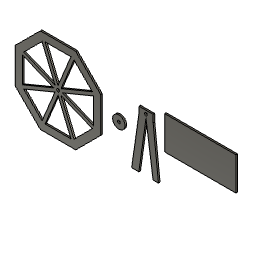
FerrisWheel2 v0 (Autodesk Fusion 360 design; units mm, degrees)
Autodesk Fusion 360 part; units mm, degrees
sketch "Sketch1" plane through (0, 0, 0) normal (0, 1, 0) x (1, 0, 0)
  line L0 (100, -41.4214) -> (100, 41.4213)
  line L1 (100, 41.4213) -> (41.4214, 100)
  line L2 (41.4214, 100) -> (-41.4213, 100)
  line L3 (-41.4213, 100) -> (-100, 41.4214)
  line L4 (-100, 41.4214) -> (-100, -41.4213)
  line L5 (-100, -41.4213) -> (-41.4214, -100)
  line L6 (-41.4214, -100) -> (41.4213, -100)
  line L7 (41.4213, -100) -> (100, -41.4214)
  line L8 (-96.5734, -44.848) -> (-100.1089, -41.3124) construction
  line L9 (-100.1089, -41.3124) -> (-100, -36.3136) construction
  line L10 (-41.4214, -100) -> (-36.4214, -100)
  line L11 (-41.4214, -100) -> (-44.9569, -96.4644)
  line L12 (-100, 41.4214) -> (-100, 36.4214)
  line L13 (-100, 41.4214) -> (-96.4644, 44.9569)
  line L14 (-41.4213, 100) -> (-36.4213, 100)
  line L15 (-41.4213, 100) -> (-44.9569, 96.4645)
  line L16 (41.4214, 100) -> (44.9569, 96.4644)
  line L17 (41.4214, 100) -> (36.4214, 100)
  line L18 (100, 41.4213) -> (100, 36.4213)
  line L19 (100, 41.4213) -> (96.4645, 44.9569)
  line L20 (100, -41.4214) -> (100, -36.4214)
  line L21 (100, -41.4214) -> (96.4644, -44.9569)
  line L22 (41.4213, -100) -> (44.9569, -96.4645)
  line L23 (41.4213, -100) -> (36.4213, -100)
  line L24 (-96.5734, -44.848) -> (100, 36.4213)
  line L25 (96.4645, 44.9569) -> (-100, -36.3136)
  line L26 (-44.9569, -96.4644) -> (36.4214, 100)
  line L27 (44.9569, 96.4644) -> (-36.4214, -100)
  line L28 (36.4213, -100) -> (-44.9569, 96.4645)
  line L29 (-36.4213, 100) -> (44.9569, -96.4645)
  line L30 (96.4644, -44.9569) -> (-100, 36.4214)
  line L31 (-96.4644, 44.9569) -> (100, -36.4214)
  circle A0 centre (0, 0) radius 4
  circle A1 centre (0, 0) radius 17.5
  line L32 (120, 49.7056) -> (49.7056, 120)
  line L33 (49.7056, 120) -> (-49.7056, 120)
  line L34 (-49.7056, 120) -> (-120, 49.7056)
  line L35 (-120, 49.7056) -> (-120, -49.7056)
  line L36 (-120, -49.7056) -> (-49.7056, -120)
  line L37 (-49.7056, -120) -> (49.7056, -120)
  line L38 (49.7056, -120) -> (120, -49.7056)
  line L39 (120, -49.7056) -> (120, 49.7056)
  line L40 (200.3187, 0) -> (200.3187, 150) construction
  line L41 (200.3187, 150) -> (220.3187, 150) construction
  line L42 (200.3187, 150) -> (180.3187, 150) construction
  line L43 (220.3187, 150) -> (235.3187, 150)
  line L44 (220.3187, -10) -> (180.3187, -10)
  line L45 (180.3187, -10) -> (180.3187, 10)
  line L46 (220.3187, 10) -> (220.3187, -10)
  line L47 (220.3187, -10) -> (180.3187, 10) construction
  line L48 (180.3187, -10) -> (220.3187, 10) construction
  line L49 (235.3187, 150) -> (220.3187, 10)
  line L50 (220.3187, 150) -> (200.3187, 10)
  line L51 (180.3187, 150) -> (200.3187, 10)
  line L52 (160, 150) -> (180.3187, 10)
  line L53 (160, 150) -> (180.3187, 150)
  line L54 (300, 0) -> (500, 0)
  line L55 (500, 0) -> (500, -93.2)
  line L56 (500, -93.2) -> (300, -93.2)
  line L57 (300, -93.2) -> (300, 0)
  point P0 (200.3187, 0)
  dimension "d5" = 100
  dimension "d6" = 5
  dimension "d7" = 5
  dimension "d10" = 5
  dimension "d11" = 5
  dimension "d12" = 5
  dimension "d13" = 5
  dimension "d14" = 5
  dimension "d15" = 5
  dimension "d16" = 5
  dimension "d17" = 5
  dimension "d18" = 5
  dimension "d19" = 5
  dimension "d20" = 5
  dimension "d21" = 5
  dimension "d22" = 5
  dimension "d23" = 5
  dimension "d25" = 8
  dimension "d26" = 35
  dimension "d28" = 120
  dimension "d42" = 150
  dimension "d43" = 20
  dimension "d44" = 20
  dimension "d45" = 15
  dimension "d46" = 40
  dimension "d47" = 20
  dimension "d48" = 200
  dimension "d49" = 93.2
  constraint coincident A0.centre A1.centre
  constraint coincident L5 L8.start
  constraint parallel L5 L8
  constraint coincident L4 L9.end
  constraint coincident L6 L10.end
  constraint coincident L5 L11.end
  constraint parallel L4 L12
  constraint parallel L3 L13
  constraint parallel L2 L14
  constraint parallel L3 L15
  constraint parallel L1 L16
  constraint parallel L2 L17
  constraint parallel L0 L18
  constraint parallel L1 L19
  constraint parallel L0 L20
  constraint parallel L7 L21
  constraint parallel L7 L22
  constraint parallel L6 L23
  constraint parallel L26 L27
  constraint parallel L0 L40
  constraint perpendicular L40 L41
  constraint perpendicular L40 L42
  constraint parallel L41 L43
  constraint horizontal L44
  constraint perpendicular L44 L45
  constraint parallel L45 L46
  constraint coincident L47 P0
  constraint coincident L48 P0
  constraint coincident P0 L40.start
  constraint horizontal L54
  constraint vertical L55
  constraint horizontal L56
  constraint vertical L57
  measures "d5" distance of A0.centre L7
  measures "d6" distance of L8.start L8.end
  measures "d7" distance of L8.end L9.end
  measures "d10" horizontal distance of L5.end L10.end
  measures "d11" distance of L5.end L11.end
  measures "d12" distance of L3.end L12.end
  measures "d13" distance of L3.end L13.end
  measures "d14" distance of L2.end L14.end
  measures "d15" distance of L2.end L15.end
  measures "d16" distance of L1.end L16.end
  measures "d17" distance of L1.end L17.end
  measures "d18" distance of L0.end L18.end
  measures "d19" distance of L0.end L19.end
  measures "d20" distance of L0.start L20.end
  measures "d21" distance of L0.start L21.end
  measures "d22" distance of L6.end L22.end
  measures "d23" distance of L6.end L23.end
  measures "d25" diameter of A0
  measures "d26" diameter of A1
  measures "d28" distance of A0.centre L39
  measures "d42" distance of P0 L40.end
  measures "d43" distance of L40.end L41.end
  measures "d44" distance of L40.end L42.end
  measures "d45" distance of L41.end L43.end
  measures "d46" distance of L45.end L46.start
  measures "d47" distance of L44.end L45.end
  measures "d48" distance of L54.start L54.end
  measures "d49" distance of L54.start L56.end
extrude "Extrude1" add sketch "Sketch1" along normal blind 4.4 contours L0 L7 L20 L21 L30 L31 A1 | L0 L1 L18 L19 L24 L25 A1 | L24 L29 L30 L31 A1 | L6 L7 L22 L23 L28 L29 A1 | L24 L25 L27 L31 A1 | L24 L27 L29 L31 | L27 L28 L29 L30 A1 | L24 L27 L29 L30 | L24 L27 L29 | L25 L27 L29 L31 | L27 L29 L31 | L24 L27 L30 | L24 L27 L28 L30 | L1 L2 L16 L17 L26 L27 A1 | L25 L26 L27 L29 A1 | L24 L25 L26 L27 L28 L29 L30 L31 | L25 L29 L31 | L5 L6 L10 L11 L26 L27 A1 | L24 L26 L27 L28 A1 | L24 L28 L30 | L25 L26 L29 L31 | L25 L26 L31 | L24 L26 L28 L30 | L26 L28 L30 | L26 L28 L29 L31 A1 | L2 L3 L14 L15 L28 L29 A1 | L25 L26 L28 | L25 L26 L28 L31 | L24 L25 L26 L30 A1 | L4 L5 L24 L25 A1 | L25 L26 L28 L30 | L25 L28 L30 L31 A1 | L3 L4 L12 L13 L30 L31 A1 | L32 L33 L34 L35 L36 L37 L38 L39 makes body 1
cylinder "CylinderPrimitive1" add diameter 35 height 4.4 placed x (1, 0, 0) y (0, 0, -1) z (0, 1, 0) at (200, 0, 0) separate body makes body 2
cylinder "CylinderPrimitive2" cut diameter 8 height 5 placed x (1, 0, 0) y (0, 0, -1) z (0, 1, 0) at (200, 0, 0) bodies 2
extrude "Extrude3" add sketch "Sketch1" against normal blind 4.4 from surface at -10 separate body contours L43 L44 L45 L46 L49 L50 L51 L52 L53 makes body 3
extrude "Extrude4" add sketch "Sketch1" along normal blind 4.4 separate body contours L54 L55 L56 L57 makes body 4
cylinder "CylinderPrimitive3" cut diameter 8 height -30 placed x (1, 0, 0) y (0, 0, -1) z (0, 1, 0) at (200, 0, 0) bodies 3
copy_body "Body->Comp1" bodies 1 removing the originals makes body 5 in component "Component"
copy_body "Body->Comp2" bodies 2 removing the originals makes body 6 in component "Component'"
copy_body "Body->Comp3" bodies 3 removing the originals makes body 7 in component "Component''"
copy_body "Body->Comp4" bodies 4 removing the originals makes body 8 in component "Component'''"
component "Component" placed x (1, 0, 0) y (0, 1, 0) z (0, 0, 1) at (0, 0, 0)
component "Component'" placed x (1, 0, 0) y (0, 1, 0) z (0, 0, 1) at (0, 0, 0)
component "Component''" placed x (1, 0, 0) y (0, 1, 0) z (0, 0, 1) at (0, 0, 0)
component "Component'''" placed x (1, 0, 0) y (0, 1, 0) z (0, 0, 1) at (0, 0, 0)
equation "outside_diameter = 100 mm"
equation "number_of_sides = 8"
equation "inner_diameter = 35 mm"
equation "distance_between = 80 mm"
equation "d5 = outside_diameter"
equation "d6 = width_of_sides"
equation "d7 = width_of_sides"
equation "width_of_sides = 5 mm"
equation "d10 = width_of_sides"
equation "d11 = width_of_sides"
equation "d12 = width_of_sides"
equation "d13 = width_of_sides"
equation "d14 = width_of_sides"
equation "d15 = width_of_sides"
equation "d16 = width_of_sides"
equation "d17 = width_of_sides"
equation "d18 = width_of_sides"
equation "d19 = width_of_sides"
equation "d20 = width_of_sides"
equation "d21 = width_of_sides"
equation "d22 = width_of_sides"
equation "d23 = width_of_sides"
equation "rotating_diameter = 8 mm"
equation "d25 = rotating_diameter"
equation "d26 = inner_diameter"
equation "holder_thickness = 20 mm"
equation "d28 = outside_diameter + holder_thickness"
equation "material_thickness = 4.4 mm"
equation "d30 = material_thickness"
equation "d36 = material_thickness"
equation "d37 = inner_diameter"
equation "d40 = rotating_diameter"
equation "height = 150 mm"
equation "d42 = height"
equation "d43 = holder_thickness"
equation "d44 = holder_thickness"
equation "d45 = width_of_sides * 3"
equation "d46 = holder_thickness * 2"
equation "d47 = holder_thickness"
equation "d48 = outside_diameter * 2"
equation "d49 = material_thickness * 3 + distance_between"
equation "d51 = -material_thickness"
equation "d53 = material_thickness"
equation "d57 = rotating_diameter"
